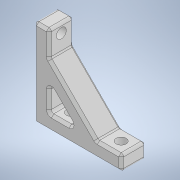
# Autodesk Inventor part: Control Board Bracket
Saved by Autodesk Inventor 2022 (Build 260153000, 153)
## iProperties
Created: 2022-04-24
Part Number: Control Board Bracket
Material: Generic
Document SubType Name: Modeling
Designer: Nick
Density: 1 g/cm^3
Appearance: Default
Author: Nick
Autodesk Inventor part; units mm, degrees
ref_plane "YZ Plane" through (0, 0, 0) normal (1, 0, 0) x (0, 1, 0)
ref_plane "XZ Plane" through (0, 0, 0) normal (0, 1, 0) x (-1, 0, 0)
ref_plane "XY Plane" through (0, 0, 0) normal (0, 0, 1) x (1, 0, 0)
sketch "Sketch1" plane through (0, 0, 0) normal (0, 0, 1) x (1, 0, 0)
  line L0 (0, 35) -> (0, 0)
  line L1 (0, 0) -> (35, 0)
  line L2 (35, 0) -> (35, 6)
  line L3 (35, 6) -> (6, 6)
  line L4 (6, 6) -> (6, 35)
  line L5 (6, 35) -> (0, 35)
  line L6 (6, 25) -> (25, 6)
  line L7 (6, 16.5147) -> (16.5147, 6)
  dimension "d0" = 6
  dimension "d1" = 35
  dimension "d5" = 45
  dimension "d6" = 10
  dimension "d24" = 6
  constraints: 16 end point, 5 perpendicular, 4 point on line, 2 parallel, 1 coincident, 1 horizontal, 1 vertical
  measures "d0" distance of L4.end L0.start
  measures "d1" distance of L0.start L0.end
  measures "d5" angle of L6 L4
  measures "d6" distance of L4.end L6.start
  measures "d24" distance between parallel lines of L6 L7
extrude "Extrusion1" add sketch "Sketch1" along normal blind 10 contours L5 L4 L3 L2 L1 L0 | L6 L3 L7 L4
sketch "Sketch2" plane through (0, 0, 0) normal (0, -1, 0) x (1, 0, 0)
  line L0 (35, 0) -> (35, 10) projected
  point P0 (0, 0)
  point P1 (30, 5)
  point P2 (10, 5)
  point P3 (35, 5)
  dimension "d7" = 5
  dimension "d8" = 20
  constraints: 2 horizontal alignment, 1 midpoint
  measures "d7" distance from line of L0 point (30, 5)
  measures "d8" distance of point (10, 5) point (30, 5)
hole "Hole1" at (30, 0, 5) at (10, 0, 5) direction (0, 1, 0) diameter 4 depth 8
sketch "Sketch3" plane through (0, 0, 0) normal (-1, 0, 0) x (0, 0, 1)
  line L0 (0, 35) -> (10, 35) projected
  line L1 (0, 0) -> (10, 0) projected
  point P0 (5, 31.5)
  point P1 (5, 35)
  dimension "d16" = 31.5
  constraints: 1 midpoint, 1 vertical alignment
  measures "d16" distance from line of L1 point (5, 31.5)
hole "Hole2" at (0, 31.5, 5) direction (1, 0, 0) diameter 4 depth 8
fillet "Fillet1" radius 1 10 edges at (0, 35, 5) (6, 35, 5) (0, 0, 5) (35, 0, 5) (35, 6, 5) (25, 6, 5) (6, 25, 5) (6, 6, 5) (6, 16.5147, 5) (16.5147, 6, 5)
chamfer "Chamfer1" distance 1 angle 45 36 edges at (0, 17.5, 10) (0.2929, 0.2929, 10) (17.5, 0, 10) (34.7071, 0.2929, 10) (35, 3, 10) (34.7071, 5.7071, 10) (29.7071, 6, 10) (25.0315, 6.0761, 10) (15.5, 15.5, 10) (6.0761, 25.0315, 10) (6, 29.7071, 10) (5.7071, 34.7071, 10) (3, 35, 10) (0.2929, 34.7071, 10) (11.2574, 11.2574, 10) (10.5503, 6, 10) (6.2929, 6.2929, 10) (6, 10.5503, 10) (6, 10.5503, 0) (11.2574, 11.2574, 0) (10.5503, 6, 0) (6.2929, 6.2929, 0) (0, 17.5, 0) (0.2929, 0.2929, 0) (17.5, 0, 0) (34.7071, 0.2929, 0) (35, 3, 0) (34.7071, 5.7071, 0) (29.7071, 6, 0) (25.0315, 6.0761, 0) (15.5, 15.5, 0) (6.0761, 25.0315, 0) (6, 29.7071, 0) (5.7071, 34.7071, 0) (3, 35, 0) (0.2929, 34.7071, 0)
body "Solid1"
